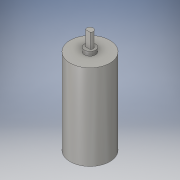
# Autodesk Inventor part: Motor
Saved by Autodesk Inventor 2016 (Build 200138000, 138)
## iProperties
Created: 2016-04-01
Part Number: Motor
Material: Generic
Document SubType Name: Modeling
Designer: amycroft3
Density: 1 g/cm^3
Appearance: Aluminum - Polished
Author: amycroft3
Autodesk Inventor part; units mm, degrees
ref_plane "YZ Plane" through (0, 0, 0) normal (1, 0, 0) x (0, 1, 0)
ref_plane "XZ Plane" through (0, 0, 0) normal (0, 1, 0) x (-1, 0, 0)
ref_plane "XY Plane" through (0, 0, 0) normal (0, 0, 1) x (1, 0, 0)
sketch "Sketch1" plane through (0, 0, 0) normal (0, 1, 0) x (-1, 0, 0)
  circle A0 centre (0, 0) radius 12.5
  dimension "d0" = 25
  constraints: 1 centre point, 1 coincident
  measures "d0" diameter of A0
extrude "Extrusion1" add sketch "Sketch1" along normal blind 53.75
sketch "Sketch2" plane through (0, 53.75, 0) normal (0, 1, 0) x (1, 0, 0)
  circle A0 centre (0, 0) radius 2
  dimension "d3" = 4
  constraints: 1 centre point, 1 coincident
  measures "d3" diameter of A0
extrude "Extrusion2" add sketch "Sketch2" along normal blind 11.938
sketch "Sketch3" plane through (0, 65.688, 0) normal (0, 1, 0) x (1, 0, 0)
  line L0 (-1.5129, -1.3081) -> (1.5129, -1.3081)
  circle A0 centre (0, 0) radius 2 projected
  arc A1 (-1.5129, -1.3081) -> (1.5129, -1.3081) centre (0, 0) ccw
  dimension "d12" = 1.3081
  constraints: 2 end point, 2 point on circle, 1 centre point, 1 coincident, 1 horizontal, 3 other
  measures "d12" distance from line of L0 point (0, 0)
extrude "Extrusion3" cut sketch "Sketch3" against normal up to surface (11.938 mm away) contours L0 A0 picked at (-0.3834, -1.4174)
sketch "Sketch4" plane through (0, 53.75, 0) normal (0, 1, 0) x (1, 0, 0)
  circle A0 centre (0, 0) radius 3.4607
  dimension "d9" = 6.9215
  constraints: 1 centre point, 1 coincident
  measures "d9" diameter of A0
extrude "Extrusion4" add sketch "Sketch4" along normal blind 2.54
body "Solid1"
